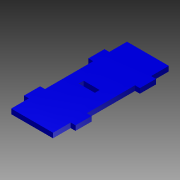
# Autodesk Inventor part: OpenROV 2.3 Dev EChassis Light Plate
Saved by Autodesk Inventor 2012 (Build 160160000, 160)
## iProperties
Created: 2012-04-29
Part Number: OpenROV 2.3 Dev EChassis Light Plate
Material: Default
Document SubType Name: Modeling
Designer: user
Density: 1 g/cm^3
Author: user
Autodesk Inventor part; units mm, degrees
ref_plane "YZ Plane" through (0, 0, 0) normal (1, 0, 0) x (0, 1, 0)
ref_plane "XZ Plane" through (0, 0, 0) normal (0, 1, 0) x (-1, 0, 0)
ref_plane "XY Plane" through (0, 0, 0) normal (0, 0, 1) x (1, 0, 0)
sketch "Sketch1" plane through (0, 0, 0) normal (0, 0, 1) x (1, 0, 0)
  line L0 (0, 0) -> (0, 10)
  line L1 (0, 10) -> (3, 10)
  line L2 (3, 10) -> (3, 40)
  line L3 (3, 40) -> (0, 40)
  line L4 (0, 40) -> (0, 50)
  line L5 (32, 50) -> (32, 40)
  line L6 (32, 40) -> (29, 40)
  line L7 (29, 40) -> (29, 10)
  line L8 (29, 10) -> (32, 10)
  line L9 (32, 10) -> (32, 0)
  line L10 (10.5, 23.5) -> (20.5, 23.5)
  line L11 (20.5, 23.5) -> (20.5, 26.5)
  line L12 (20.5, 26.5) -> (10.5, 26.5)
  line L13 (10.5, 26.5) -> (10.5, 23.5)
  line L14 (3, 50) -> (3, 61)
  line L15 (3, 61) -> (29, 61)
  line L16 (29, 61) -> (29, 50)
  line L17 (3, 0) -> (3, -11)
  line L18 (3, -11) -> (29, -11)
  line L19 (29, -11) -> (29, 0)
  line L20 (0, 50) -> (3, 50)
  line L21 (29, 50) -> (32, 50)
  line L22 (32, 0) -> (29, 0)
  line L23 (3, 0) -> (0, 0)
  dimension "d19" = 10
  dimension "d20" = 3
  dimension "d22" = 10
  dimension "d23" = 3
  dimension "d24" = 30
  dimension "d25" = 3
  dimension "d26" = 10
  dimension "d27" = 32
  dimension "d28" = 10
  dimension "d29" = 3
  dimension "d30" = 3
  dimension "d31" = 10
  dimension "d32" = 7.5
  dimension "d35" = 30
  dimension "d36" = 72
  dimension "d39" = 34.5
  dimension "d40" = 26
  dimension "d41" = 26
  dimension "d42" = 11
  dimension "d43" = 11
  constraints: 48 end point, 16 parallel, 8 perpendicular, 2 collinear, 1 vertical
  measures "d19" distance of L11.end L12.end
  measures "d20" distance of L10.end L11.end
  measures "d22" distance of L0.start L0.end
  measures "d23" distance of L0.end L1.end
  measures "d24" distance of L1.end L2.end
  measures "d25" distance of L2.end L3.end
  measures "d26" distance of L3.end L4.end
  measures "d27" distance of L4.end L5.start
  measures "d28" distance of L5.start L5.end
  measures "d29" distance of L5.end L6.end
  measures "d30" distance of L7.end L8.end
  measures "d31" distance of L8.end L9.end
  measures "d32" distance between parallel lines of L2 L13
  measures "d35" distance of L6.end L7.end
  measures "d36" distance between parallel lines of L18 L15
  measures "d39" distance between parallel lines of L18 L10
  measures "d40" distance of L14.end L15.end
  measures "d41" distance of L17.end L18.end
  measures "d42" distance between parallel lines of L18 L23
  measures "d43" distance between parallel lines of L21 L15
extrude "Extrusion1" add sketch "Sketch1" along normal blind 3
body "Solid1"
